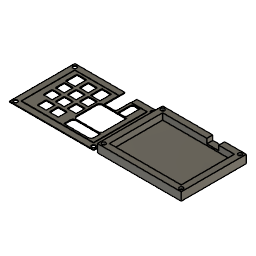
hackpad-case (Autodesk Fusion 360 design; units mm, degrees)
part number: 2026-01-27-21-45-44-218
Autodesk Fusion 360 part; units mm, degrees
sketch "Sketch1" plane through (0, 0, 0) normal (0, 0, 1) x (1, 0, 0)
  line L0 (56.89, -42.155) -> (-56.89, -42.155)
  line L1 (-56.89, -42.155) -> (-56.89, 42.155)
  line L2 (-56.89, 42.155) -> (56.89, 42.155)
  line L3 (56.89, 42.155) -> (56.89, -42.155)
  line L4 (56.89, -42.155) -> (-56.89, 42.155) construction
  line L5 (-56.89, -42.155) -> (56.89, 42.155) construction
  line L6 (66.39, 51.655) -> (-66.39, 51.655)
  line L7 (-66.39, 51.655) -> (-66.39, -51.655)
  line L8 (-66.39, -51.655) -> (66.39, -51.655)
  line L9 (66.39, -51.655) -> (66.39, 51.655)
  line L10 (66.39, 51.655) -> (-66.39, -51.655) construction
  line L11 (-66.39, 51.655) -> (66.39, -51.655) construction
  circle A0 centre (61.39, 46.655) radius 1.7
  circle A1 centre (61.39, -46.655) radius 1.7
  circle A2 centre (-61.39, -46.655) radius 1.7
  circle A3 centre (-61.39, 46.655) radius 1.7
  circle A4 centre (61.39, 46.655) radius 3
  circle A5 centre (61.39, -46.655) radius 3
  circle A6 centre (-61.39, -46.655) radius 3
  circle A7 centre (-61.39, 46.655) radius 3
  dimension "d1" = 113.78
  dimension "d2" = 84.31
  dimension "d7" = 3.4
  dimension "d8" = 5
  dimension "d9" = 5
  dimension "d10" = 9.5
  dimension "d11" = 9.5
  dimension "d12" = 9.5
  dimension "d13" = 3.4
  dimension "d14" = 5
  dimension "d15" = 5
  dimension "d16" = 3.4
  dimension "d17" = 5
  dimension "d18" = 5
  dimension "d19" = 3.4
  dimension "d20" = 5
  dimension "d21" = 5
  dimension "d22" = 6
  dimension "d23" = 6
  dimension "d24" = 6
  dimension "d25" = 6
  constraint horizontal L0
  constraint perpendicular L0 L1
  constraint parallel L0 L2
  constraint parallel L1 L3
  constraint coincident L4 origin
  constraint coincident L5 origin
  constraint horizontal L6
  constraint perpendicular L6 L7
  constraint parallel L6 L8
  constraint parallel L7 L9
  constraint coincident L10 origin
  constraint coincident L11 origin
  constraint concentric A0 A4
  constraint concentric A1 A5
  constraint concentric A2 A6
  constraint concentric A3 A7
  measures "d1" distance of L1.end L2.end
  measures "d2" distance of L0.end L1.end
  measures "d7" diameter of A0
  measures "d8" distance of L9 A0.centre
  measures "d9" distance of L6 A0.centre
  measures "d10" distance of L2 L6
  measures "d11" distance of L0 L8
  measures "d12" distance of L3 L9
  measures "d13" diameter of A1
  measures "d14" distance of L8 A1.centre
  measures "d15" distance of L9 A1.centre
  measures "d16" diameter of A2
  measures "d17" distance of L8 A2.centre
  measures "d18" distance of L7 A2.centre
  measures "d19" diameter of A3
  measures "d20" distance of L6 A3.centre
  measures "d21" distance of L7 A3.centre
  measures "d22" diameter of A4
  measures "d23" diameter of A5
  measures "d24" diameter of A6
  measures "d25" diameter of A7
extrude "Extrude1" add sketch "Sketch1" along normal blind 9.9 from surface at 3.1 contours A4 | A5 | A6 | A7 makes body 1 at (-58.3937, -46.8045, 9.7) makes body 2 at (63.9499, -48.2193, 9.7) makes body 3 at (-63.9499, 48.2193, 9.7) makes body 4 at (58.3937, 46.5055, 9.7)
extrude "Extrude2" add sketch "Sketch1" along normal blind 13 contours L6 L7 L8 L9 bodies 1 2 3 4
extrude "Extrude3" add sketch "Sketch1" along normal blind 3 contours L0 L1 L2 L3 bodies 1
sketch "Sketch2" plane through (0, 0, 13) normal (0, 0, 1) x (-1, 0, 0)
  circle A0 centre (61.39, 46.655) radius 1.7
  circle A1 centre (-61.39, -46.655) radius 1.7
  line L0 (56.89, -42.155) -> (-56.89, -42.155)
  line L1 (-56.89, -42.155) -> (-56.89, 42.155)
  line L2 (-56.89, 42.155) -> (56.89, 42.155)
  line L3 (56.89, 42.155) -> (56.89, -42.155)
  line L4 (-66.39, 51.655) -> (-66.39, -51.655)
  line L5 (-66.39, -51.655) -> (66.39, -51.655)
  line L6 (66.39, -51.655) -> (66.39, 51.655)
  line L7 (66.39, 51.655) -> (-66.39, 51.655)
  circle A2 centre (-61.39, 46.655) radius 1.7
  circle A3 centre (61.39, -46.655) radius 1.7
  line L8 (-12.076, -51.655) -> (-12.076, -42.155)
  line L9 (-30.576, -51.655) -> (-30.576, -42.155)
  line L10 (-66.39, 51.655) -> (-66.39, -51.655)
  line L11 (-56.89, -42.155) -> (-56.89, 42.155)
  dimension "d33" = 18.5
  dimension "d35" = 26.314
  constraint coincident L5 L8.start
  constraint coincident L0 L8.end
  constraint perpendicular L0 L8
  constraint coincident L5 L9.start
  constraint coincident L0 L9.end
  constraint perpendicular L5 L9
  measures "d33" distance of L8 L9
  measures "d35" distance of L9 L11
extrude "Extrude4" cut sketch "Sketch2" against normal blind 7.5 contours L0 L5 L8 L9 bodies 1
sketch "plate-2026-01-28T03_03_28.937Z" plane through (0, 0, 0) normal (0, 0, 1) x (1, 0, 0)
  line L0 (-162.925, -2.525) -> (-149.925, -2.525)
  line L1 (-162.925, -16.525) -> (-149.925, -16.525)
  line L2 (-163.425, -3.025) -> (-163.425, -16.025)
  line L3 (-149.425, -3.025) -> (-149.425, -16.025)
  arc A0 (-162.925, -2.525) -> (-163.425, -3.025) centre (-162.925, -3.025) ccw
  arc A1 (-149.425, -3.025) -> (-149.925, -2.525) centre (-149.925, -3.025) ccw
  arc A2 (-163.425, -16.025) -> (-162.925, -16.525) centre (-162.925, -16.025) ccw
  arc A3 (-149.925, -16.525) -> (-149.425, -16.025) centre (-149.925, -16.025) ccw
  line L4 (-181.975, -21.575) -> (-168.975, -21.575)
  line L5 (-181.975, -35.575) -> (-168.975, -35.575)
  line L6 (-182.475, -22.075) -> (-182.475, -35.075)
  line L7 (-168.475, -22.075) -> (-168.475, -35.075)
  arc A4 (-181.975, -21.575) -> (-182.475, -22.075) centre (-181.975, -22.075) ccw
  arc A5 (-168.475, -22.075) -> (-168.975, -21.575) centre (-168.975, -22.075) ccw
  arc A6 (-182.475, -35.075) -> (-181.975, -35.575) centre (-181.975, -35.075) ccw
  arc A7 (-168.975, -35.575) -> (-168.475, -35.075) centre (-168.975, -35.075) ccw
  line L8 (-162.925, -21.575) -> (-149.925, -21.575)
  line L9 (-162.925, -35.575) -> (-149.925, -35.575)
  line L10 (-163.425, -22.075) -> (-163.425, -35.075)
  line L11 (-149.425, -22.075) -> (-149.425, -35.075)
  arc A8 (-162.925, -21.575) -> (-163.425, -22.075) centre (-162.925, -22.075) ccw
  arc A9 (-149.425, -22.075) -> (-149.925, -21.575) centre (-149.925, -22.075) ccw
  arc A10 (-163.425, -35.075) -> (-162.925, -35.575) centre (-162.925, -35.075) ccw
  arc A11 (-149.925, -35.575) -> (-149.425, -35.075) centre (-149.925, -35.075) ccw
  line L12 (-143.875, -21.575) -> (-130.875, -21.575)
  line L13 (-143.875, -35.575) -> (-130.875, -35.575)
  line L14 (-144.375, -22.075) -> (-144.375, -35.075)
  line L15 (-130.375, -22.075) -> (-130.375, -35.075)
  arc A12 (-143.875, -21.575) -> (-144.375, -22.075) centre (-143.875, -22.075) ccw
  arc A13 (-130.375, -22.075) -> (-130.875, -21.575) centre (-130.875, -22.075) ccw
  arc A14 (-144.375, -35.075) -> (-143.875, -35.575) centre (-143.875, -35.075) ccw
  arc A15 (-130.875, -35.575) -> (-130.375, -35.075) centre (-130.875, -35.075) ccw
  line L16 (-181.975, -40.625) -> (-168.975, -40.625)
  line L17 (-181.975, -54.625) -> (-168.975, -54.625)
  line L18 (-182.475, -41.125) -> (-182.475, -54.125)
  line L19 (-168.475, -41.125) -> (-168.475, -54.125)
  arc A16 (-181.975, -40.625) -> (-182.475, -41.125) centre (-181.975, -41.125) ccw
  arc A17 (-168.475, -41.125) -> (-168.975, -40.625) centre (-168.975, -41.125) ccw
  arc A18 (-182.475, -54.125) -> (-181.975, -54.625) centre (-181.975, -54.125) ccw
  arc A19 (-168.975, -54.625) -> (-168.475, -54.125) centre (-168.975, -54.125) ccw
  line L20 (-162.925, -40.625) -> (-149.925, -40.625)
  line L21 (-162.925, -54.625) -> (-149.925, -54.625)
  line L22 (-163.425, -41.125) -> (-163.425, -54.125)
  line L23 (-149.425, -41.125) -> (-149.425, -54.125)
  arc A20 (-162.925, -40.625) -> (-163.425, -41.125) centre (-162.925, -41.125) ccw
  arc A21 (-149.425, -41.125) -> (-149.925, -40.625) centre (-149.925, -41.125) ccw
  arc A22 (-163.425, -54.125) -> (-162.925, -54.625) centre (-162.925, -54.125) ccw
  arc A23 (-149.925, -54.625) -> (-149.425, -54.125) centre (-149.925, -54.125) ccw
  line L24 (-143.875, -40.625) -> (-130.875, -40.625)
  line L25 (-143.875, -54.625) -> (-130.875, -54.625)
  line L26 (-144.375, -41.125) -> (-144.375, -54.125)
  line L27 (-130.375, -41.125) -> (-130.375, -54.125)
  arc A24 (-143.875, -40.625) -> (-144.375, -41.125) centre (-143.875, -41.125) ccw
  arc A25 (-130.375, -41.125) -> (-130.875, -40.625) centre (-130.875, -41.125) ccw
  arc A26 (-144.375, -54.125) -> (-143.875, -54.625) centre (-143.875, -54.125) ccw
  arc A27 (-130.875, -54.625) -> (-130.375, -54.125) centre (-130.875, -54.125) ccw
  circle A28 centre (-191.875, 4.4557) radius 1.7
  circle A29 centre (-79.875, -81.8599) radius 1.7
  line L28 (-196.875, 10.1401) -> (-196.875, -86.8599)
  line L29 (-196.875, -86.8599) -> (-74.875, -86.8599)
  line L30 (-74.875, -86.8599) -> (-74.875, 9.4557)
  line L31 (-74.875, 9.4557) -> (-109.2354, 9.4557)
  line L32 (-109.2354, -0.0443) -> (-84.2214, -0.0179)
  line L33 (-84.2214, -0.0179) -> (-84.2214, -78.5291)
  line L34 (-84.2214, -78.5291) -> (-187.375, -78.5291)
  line L35 (-187.375, -78.5291) -> (-187.375, -0.0443)
  line L36 (-187.375, -0.0443) -> (-107.2527, -0.0443)
  circle A30 centre (-79.875, 4.4557) radius 1.7
  circle A31 centre (-191.875, -81.8599) radius 1.7
  line L37 (-187.375, -0.0443) -> (-187.375, -78.5291)
  line L38 (-187.375, -78.5291) -> (-84.2214, -78.5291)
  line L39 (-84.2214, -78.5291) -> (-84.2214, -0.0179)
  line L40 (-196.875, 9.4557) -> (-109.2354, 9.4557)
  line L41 (-109.2354, -0.0443) -> (-107.2527, -0.0443)
  circle A32 centre (-191.875, 4.4557) radius 3
  circle A33 centre (-191.875, -81.8599) radius 3
  circle A34 centre (-79.875, -81.8599) radius 3
  circle A35 centre (-79.875, 4.4557) radius 3
  line L42 (-123.3934, -26.7131) -> (-85.9914, -26.7131)
  line L43 (-85.9914, -26.7131) -> (-85.9914, -53.0661)
  line L44 (-89.9914, -57.0661) -> (-122.3934, -57.0661)
  line L45 (-127.3934, -52.0661) -> (-127.3934, -30.7131)
  line L46 (-124.3934, -61.2571) -> (-85.9914, -61.2571)
  line L47 (-85.9914, -61.2571) -> (-85.9914, -70.3221)
  line L48 (-88.9914, -73.3221) -> (-127.3934, -73.3221)
  line L49 (-127.3934, -73.3221) -> (-127.3934, -64.2571)
  line L50 (-196.875, 10.1401) -> (-196.875, 9.4557)
  arc A36 (-127.3934, -52.0661) -> (-122.3934, -57.0661) centre (-122.3934, -52.0661) ccw
  line L51 (-123.3934, -26.7131) -> (-127.3934, -30.7131)
  line L52 (-85.9914, -53.0661) -> (-89.9914, -57.0661)
  line L53 (-127.3934, -64.2571) -> (-124.3934, -61.2571)
  line L54 (-85.9914, -70.3221) -> (-88.9914, -73.3221)
  line L55 (-98.0014, -2.3043) -> (-92.2714, -2.3043)
  line L56 (-90.2714, -4.3043) -> (-90.2714, -23.1243)
  line L57 (-90.2714, -23.1243) -> (-98.0014, -23.1243)
  line L58 (-100.0014, -21.1243) -> (-100.0014, -4.3043)
  line L59 (-121.1354, -0.3901) -> (-105.3354, -0.3901)
  line L60 (-105.3354, -0.3901) -> (-105.3354, -19.6081)
  line L61 (-107.3354, -21.6081) -> (-120.1354, -21.6081)
  line L62 (-123.1354, -18.6081) -> (-123.1354, -2.3901)
  line L63 (-119.2354, -0.0268) -> (-119.2354, 9.4557)
  line L64 (-109.2354, -0.0443) -> (-109.2354, 9.4557)
  arc A37 (-121.1354, -0.3901) -> (-123.1354, -2.3901) centre (-121.1354, -2.3901) ccw
  arc A38 (-107.3354, -21.6081) -> (-105.3354, -19.6081) centre (-107.3354, -19.6081) ccw
  arc A39 (-90.2714, -4.3043) -> (-92.2714, -2.3043) centre (-92.2714, -4.3043) ccw
  arc A40 (-100.0014, -21.1243) -> (-98.0014, -23.1243) centre (-98.0014, -21.1243) ccw
  line L65 (-123.1354, -18.6081) -> (-123.1354, -21.6081)
  line L66 (-123.1354, -21.6081) -> (-120.1354, -21.6081)
  line L67 (-98.0014, -2.3043) -> (-100.0014, -2.3043)
  line L68 (-100.0014, -2.3043) -> (-100.0014, -4.3043)
  line L69 (-119.2354, -0.0268) -> (-119.2354, -0.3901)
  line L70 (-109.2354, -0.0443) -> (-109.2354, -0.3901)
  point P0 (-79.875, -81.8599)
  point P1 (-190.0693, -81.8599)
  point P2 (-190.0693, 5.1401)
  point P3 (-78.0693, 5.1401)
  point P4 (-127.3934, -26.7131)
  point P5 (-85.9914, -57.0661)
  point P6 (-127.3934, -57.0661)
  point P7 (-127.3934, -61.2571)
  point P8 (-85.9914, -73.3221)
  point P9 (-100.0014, -2.3043)
  point P10 (-90.2714, -2.3043)
  point P11 (-100.0014, -23.1243)
  point P12 (-123.1354, -0.3901)
  point P13 (-123.1354, -21.6081)
  dimension "d44" = 5.05
  dimension "d53" = 6
  dimension "d54" = 6
  dimension "d55" = 6
  dimension "d56" = 6
  dimension "d57" = 9.5
  dimension "d63" = 97
  dimension "d64" = 9.5
  dimension "d65" = 9.5
  dimension "d66" = 4.9
  dimension "d71" = 30.353
  dimension "d72" = 12.065
  dimension "d73" = 1.77
  dimension "d74" = 1.77
  dimension "d75" = 41.402
  dimension "d76" = 41.402
  dimension "d77" = 4.191
  dimension "d78" = 5.207
  dimension "d79" = 3.4
  dimension "d80" = 5
  dimension "d81" = 5
  dimension "d83" = 122
  dimension "d84" = 5
  dimension "d85" = 5
  dimension "d86" = 5
  dimension "d87" = 5
  dimension "d88" = 5
  dimension "d89" = 3.4
  dimension "d90" = 5
  dimension "d91" = 5
  dimension "d93" = 4
  dimension "d94" = 4
  dimension "d95" = 4
  dimension "d96" = 3
  dimension "d97" = 3
  dimension "d98" = 3
  dimension "d99" = 3
  dimension "d100" = 9.73
  dimension "d101" = 20.82
  dimension "d102" = 6.05
  dimension "d103" = 2.28
  dimension "d104" = 17.8
  dimension "d105" = 21.218
  dimension "d106" = 5.334
  dimension "d107" = 0.35
  dimension "d109" = 10
  dimension "d110" = 3.9
  dimension "d111" = 3.9
  dimension "d112" = 2
  dimension "d113" = 2
  dimension "d114" = 2
  dimension "d115" = 3
  dimension "d116" = 3
  dimension "d117" = 2
  dimension "d118" = 2
  constraint parallel L31 L40
  constraint parallel L36 L41
  constraint concentric A28 A32
  constraint concentric A31 A33
  constraint coincident P0 A29.centre
  constraint concentric A30 A35
  constraint vertical L39
  constraint horizontal L42
  constraint vertical L43
  constraint horizontal L44
  constraint vertical L45
  constraint horizontal L46
  constraint vertical L47
  constraint horizontal L48
  constraint vertical L49
  constraint perpendicular L40 L50
  constraint horizontal L29
  constraint vertical L30
  constraint horizontal L31
  constraint horizontal L34
  constraint concentric A29 A34
  constraint coincident P6 L45
  constraint coincident P6 L44
  constraint tangent L45 A36
  constraint tangent L44 A36
  constraint coincident P4 L42
  constraint coincident P4 L45
  constraint coincident P5 L43
  constraint coincident P5 L44
  constraint coincident P7 L49
  constraint coincident P7 L46
  constraint coincident P8 L47
  constraint coincident P8 L48
  constraint horizontal L55
  constraint vertical L56
  constraint horizontal L57
  constraint vertical L58
  constraint horizontal L59
  constraint vertical L60
  constraint horizontal L61
  constraint vertical L62
  constraint coincident L40 L63.end
  constraint perpendicular L40 L63
  constraint coincident P12 L59
  constraint coincident P12 L62
  constraint tangent L59 A37
  constraint tangent L62 A37
  constraint tangent L60 A38
  constraint tangent L61 A38
  constraint coincident P10 L55
  constraint coincident P10 L56
  constraint tangent L55 A39
  constraint tangent L56 A39
  constraint coincident P11 L57
  constraint coincident P11 L58
  constraint tangent L57 A40
  constraint tangent L58 A40
  constraint equal A39 A40
  constraint coincident P13 L62
  constraint coincident P13 L61
  constraint coincident P9 L55
  constraint coincident P9 L58
  constraint coincident P13 L65.end
  constraint coincident P9 L67.end
  constraint coincident L59 L69.end
  constraint perpendicular L59 L69
  constraint coincident L59 L70.end
  constraint perpendicular L59 L70
  measures "d44" distance of L9 L20
  measures "d53" diameter of A32
  measures "d54" diameter of A33
  measures "d55" diameter of A34
  measures "d56" diameter of A35
  measures "d57" distance of L31.end L32.start
  measures "d63" distance of L28.start L28.end
  measures "d64" distance of L28 L37
  measures "d65" distance of L40 L41
  measures "d66" distance of L6 L37
  measures "d71" distance of P4 P6
  measures "d72" distance of P7 L48.end
  measures "d73" distance of L39 L43
  measures "d74" distance of L33 L47
  measures "d75" distance of P8 L48.end
  measures "d76" distance of P5 P6
  measures "d77" distance of L44 L46
  measures "d78" vertical distance of L33.end P8
  measures "d79" diameter of A31
  measures "d80" distance of L28 A31.centre
  measures "d81" distance of L29 A31.centre
  measures "d83" distance of L28.end L29.end
  measures "d84" distance of A28.centre L40
  measures "d85" distance of A28.centre L28
  measures "d86" distance of L31 A30.centre
  measures "d87" distance of L30 A30.centre
  measures "d88" distance of P0 L30
  measures "d89" diameter of A29
  measures "d90" distance of P0 L29
  measures "d91" radius of A36
  measures "d93" distance of P4 L45.end
  measures "d94" distance of P5 L43.end
  measures "d95" distance of P5 L44.start
  measures "d96" distance of P7 L49.end
  measures "d97" distance of P7 L46.start
  measures "d98" distance of P8 L47.end
  measures "d99" distance of P8 L48.start
  measures "d100" distance of P9 P10
  measures "d101" distance of P9 P11
  measures "d102" distance of L33 L56
  measures "d103" distance of L32 P10
  measures "d104" distance of P12 L59.end
  measures "d105" distance of P12 P13
  measures "d106" distance of L58 L60
  measures "d107" distance of L32 L59.end
  measures "d109" horizontal distance of L32.start L63.start
  measures "d110" horizontal distance of L32.start L59.end
  measures "d111" horizontal distance of P12 L63.start
  measures "d112" radius of A37
  measures "d113" radius of A38
  measures "d114" radius of A39
  measures "d115" distance of P13 L62.start
  measures "d116" distance of P13 L61.end
  measures "d117" distance of P9 L55.start
  measures "d118" distance of P9 L58.end
extrude "Extrude7" add 1 faces at (24.4093, 45.3217, 5.5) along direction (0, 0, 1) blind 7.5 on bodies 1 bodies 1
other "Base Mesh Feature1"
sketch "Sketch4" plane through (0, 0, 13) normal (0, 0, 1) x (-1, 0, 0)
  line L0 (56.89, -42.155) -> (-56.89, -42.155)
  line L1 (-56.89, -42.155) -> (-56.89, 42.155)
  line L2 (-56.89, 42.155) -> (56.89, 42.155)
  line L3 (56.89, 42.155) -> (56.89, -42.155)
  circle A0 centre (61.39, -46.655) radius 1.7
  circle A1 centre (-61.39, 46.655) radius 1.7
  line L4 (-66.39, -51.655) -> (66.39, -51.655)
  line L5 (66.39, -51.655) -> (66.39, 51.655)
  line L6 (66.39, 51.655) -> (-66.39, 51.655)
  line L7 (-66.39, 51.655) -> (-66.39, -51.655)
  circle A2 centre (-61.39, -46.655) radius 1.7
  circle A3 centre (61.39, 46.655) radius 1.7
  line L8 (56.89, -42.155) -> (-56.89, -42.155)
  line L9 (-56.89, -42.155) -> (-56.89, 42.155)
  line L10 (-56.89, 42.155) -> (56.89, 42.155)
  line L11 (56.89, 42.155) -> (56.89, -42.155)
  circle A4 centre (61.39, -46.655) radius 1.7
  circle A5 centre (61.39, -46.655) radius 3
  circle A6 centre (61.39, 46.655) radius 1.7
  circle A7 centre (61.39, 46.655) radius 3
  circle A8 centre (-61.39, 46.655) radius 1.7
  circle A9 centre (-61.39, 46.655) radius 3
  circle A10 centre (-61.39, -46.655) radius 1.7
  circle A11 centre (-61.39, -46.655) radius 3
  dimension "d125" = 6
  dimension "d126" = 6
  dimension "d127" = 6
  dimension "d128" = 6
  constraint horizontal L8
  constraint vertical L9
  constraint horizontal L10
  constraint vertical L11
  constraint coincident L1.end L2.start
  constraint coincident L0.start L3.end
  constraint concentric A0 A4
  constraint concentric A4 A5
  constraint concentric A3 A6
  constraint concentric A6 A7
  constraint concentric A1 A8
  constraint concentric A8 A9
  constraint concentric A2 A10
  constraint concentric A10 A11
  measures "d125" diameter of A5
  measures "d126" diameter of A7
  measures "d127" diameter of A9
  measures "d128" diameter of A11
sketch "plate-2026-01-28T03_03_28.937Z (1)" plane through (0, 0, 13) normal (0, 0, 1) x (1, 0, 0)
  line L0 (111.5924, 36.2585) -> (124.5924, 36.2585)
  line L1 (111.5924, 22.2585) -> (124.5924, 22.2585)
  line L2 (111.0924, 35.7585) -> (111.0924, 22.7585)
  line L3 (125.0924, 35.7585) -> (125.0924, 22.7585)
  arc A0 (111.5924, 36.2585) -> (111.0924, 35.7585) centre (111.5924, 35.7585) ccw
  arc A1 (125.0924, 35.7585) -> (124.5924, 36.2585) centre (124.5924, 35.7585) ccw
  arc A2 (111.0924, 22.7585) -> (111.5924, 22.2585) centre (111.5924, 22.7585) ccw
  arc A3 (124.5924, 22.2585) -> (125.0924, 22.7585) centre (124.5924, 22.7585) ccw
  line L4 (92.5424, 17.2085) -> (105.5424, 17.2085)
  line L5 (92.5424, 3.2085) -> (105.5424, 3.2085)
  line L6 (92.0424, 16.7085) -> (92.0424, 3.7085)
  line L7 (106.0424, 16.7085) -> (106.0424, 3.7085)
  arc A4 (92.5424, 17.2085) -> (92.0424, 16.7085) centre (92.5424, 16.7085) ccw
  arc A5 (106.0424, 16.7085) -> (105.5424, 17.2085) centre (105.5424, 16.7085) ccw
  arc A6 (92.0424, 3.7085) -> (92.5424, 3.2085) centre (92.5424, 3.7085) ccw
  arc A7 (105.5424, 3.2085) -> (106.0424, 3.7085) centre (105.5424, 3.7085) ccw
  line L8 (111.5924, 17.2085) -> (124.5924, 17.2085)
  line L9 (111.5924, 3.2085) -> (124.5924, 3.2085)
  line L10 (111.0924, 16.7085) -> (111.0924, 3.7085)
  line L11 (125.0924, 16.7085) -> (125.0924, 3.7085)
  arc A8 (111.5924, 17.2085) -> (111.0924, 16.7085) centre (111.5924, 16.7085) ccw
  arc A9 (125.0924, 16.7085) -> (124.5924, 17.2085) centre (124.5924, 16.7085) ccw
  arc A10 (111.0924, 3.7085) -> (111.5924, 3.2085) centre (111.5924, 3.7085) ccw
  arc A11 (124.5924, 3.2085) -> (125.0924, 3.7085) centre (124.5924, 3.7085) ccw
  line L12 (130.6424, 17.2085) -> (143.6424, 17.2085)
  line L13 (130.6424, 3.2085) -> (143.6424, 3.2085)
  line L14 (130.1424, 16.7085) -> (130.1424, 3.7085)
  line L15 (144.1424, 16.7085) -> (144.1424, 3.7085)
  arc A12 (130.6424, 17.2085) -> (130.1424, 16.7085) centre (130.6424, 16.7085) ccw
  arc A13 (144.1424, 16.7085) -> (143.6424, 17.2085) centre (143.6424, 16.7085) ccw
  arc A14 (130.1424, 3.7085) -> (130.6424, 3.2085) centre (130.6424, 3.7085) ccw
  arc A15 (143.6424, 3.2085) -> (144.1424, 3.7085) centre (143.6424, 3.7085) ccw
  line L16 (92.5424, -1.8415) -> (105.5424, -1.8415)
  line L17 (92.5424, -15.8415) -> (105.5424, -15.8415)
  line L18 (92.0424, -2.3415) -> (92.0424, -15.3415)
  line L19 (106.0424, -2.3415) -> (106.0424, -15.3415)
  arc A16 (92.5424, -1.8415) -> (92.0424, -2.3415) centre (92.5424, -2.3415) ccw
  arc A17 (106.0424, -2.3415) -> (105.5424, -1.8415) centre (105.5424, -2.3415) ccw
  arc A18 (92.0424, -15.3415) -> (92.5424, -15.8415) centre (92.5424, -15.3415) ccw
  arc A19 (105.5424, -15.8415) -> (106.0424, -15.3415) centre (105.5424, -15.3415) ccw
  line L20 (111.5924, -1.8415) -> (124.5924, -1.8415)
  line L21 (111.5924, -15.8415) -> (124.5924, -15.8415)
  line L22 (111.0924, -2.3415) -> (111.0924, -15.3415)
  line L23 (125.0924, -2.3415) -> (125.0924, -15.3415)
  arc A20 (111.5924, -1.8415) -> (111.0924, -2.3415) centre (111.5924, -2.3415) ccw
  arc A21 (125.0924, -2.3415) -> (124.5924, -1.8415) centre (124.5924, -2.3415) ccw
  arc A22 (111.0924, -15.3415) -> (111.5924, -15.8415) centre (111.5924, -15.3415) ccw
  arc A23 (124.5924, -15.8415) -> (125.0924, -15.3415) centre (124.5924, -15.3415) ccw
  line L24 (130.6424, -1.8415) -> (143.6424, -1.8415)
  line L25 (130.6424, -15.8415) -> (143.6424, -15.8415)
  line L26 (130.1424, -2.3415) -> (130.1424, -15.3415)
  line L27 (144.1424, -2.3415) -> (144.1424, -15.3415)
  arc A24 (130.6424, -1.8415) -> (130.1424, -2.3415) centre (130.6424, -2.3415) ccw
  arc A25 (144.1424, -2.3415) -> (143.6424, -1.8415) centre (143.6424, -2.3415) ccw
  arc A26 (130.1424, -15.3415) -> (130.6424, -15.8415) centre (130.6424, -15.3415) ccw
  arc A27 (143.6424, -15.8415) -> (144.1424, -15.3415) centre (143.6424, -15.3415) ccw
  line L28 (121.2182, -34.8915) -> (134.2185, -34.8915)
  arc A28 (134.2185, -34.8915) -> (134.7185, -34.3915) centre (134.2185, -34.3915) ccw
  arc A29 (134.7185, -21.3915) -> (134.2185, -20.8915) centre (134.2185, -21.3915) ccw
  arc A30 (120.6174, -34.3915) -> (121.2182, -34.8915) centre (121.1587, -34.352) ccw
  arc A31 (121.2182, -20.8915) -> (120.6174, -21.3914) centre (121.1587, -21.4309) ccw
  line L29 (120.6174, -21.3914) -> (120.6174, -34.3915)
  line L30 (134.7185, -21.3915) -> (134.7185, -34.3915)
  line L31 (121.2182, -20.8915) -> (134.2185, -20.8915)
  line L32 (114.9665, -34.8915) -> (101.9662, -34.8915)
  arc A32 (115.5674, -21.3914) -> (114.9665, -20.8915) centre (115.026, -21.4309) ccw
  line L33 (101.4662, -21.3915) -> (101.4662, -34.3915)
  line L34 (114.9665, -20.8915) -> (101.9662, -20.8915)
  arc A33 (101.9662, -20.8915) -> (101.4662, -21.3915) centre (101.9662, -21.3915) ccw
  arc A34 (114.9665, -34.8915) -> (115.5674, -34.3915) centre (115.026, -34.352) ccw
  line L35 (115.5674, -21.3914) -> (115.5674, -34.3915)
  arc A35 (101.4662, -34.3915) -> (101.9662, -34.8915) centre (101.9662, -34.3915) ccw
  circle A36 centre (61.39, 46.655) radius 1.7
  circle A37 centre (61.39, -46.655) radius 1.7
  line L36 (-56.89, 42.155) -> (56.89, 42.155)
  dimension "d130" = 5.05
  dimension "d134" = 5.05
  dimension "d135" = 5.8965
  measures "d130" distance of L21 L31
  measures "d134" distance of L29 L35
  measures "d135" distance of L0 L36
sketch "Sketch6" plane through (0, 0, 13) normal (0, 0, 1) x (1, 0, 0)
  line L0 (197.7016, -41.9833) -> (83.1186, -41.9833)
  line L1 (83.1186, -41.9833) -> (83.1186, 42.8484)
  line L2 (83.1186, 42.8484) -> (197.7016, 42.8484)
  line L3 (197.7016, 42.8484) -> (197.7016, -41.9833)
  line L4 (153.1976, -24.3309) -> (191.1976, -24.3309)
  line L5 (191.1976, -24.3309) -> (191.1976, -34.3309)
  line L6 (186.1976, -39.3309) -> (148.1976, -39.3309)
  line L7 (148.1976, -39.3309) -> (148.1976, -29.3309)
  line L8 (150.6321, 17.4739) -> (190.6321, 17.4739)
  line L9 (190.6321, 17.4739) -> (190.6321, -20.5261)
  line L10 (187.6321, -23.5261) -> (152.6321, -23.5261)
  line L11 (147.6321, -18.5261) -> (147.6321, 14.4739)
  line L12 (179, 41) -> (188, 41)
  line L13 (188, 41) -> (188, 21.5)
  line L14 (185, 18.5) -> (176, 18.5)
  line L15 (176, 18.5) -> (176, 38)
  line L16 (153.3081, 42.8484) -> (172, 42.8484)
  line L17 (172, 42.8484) -> (172, 22)
  line L18 (169, 19) -> (153.3081, 19)
  line L19 (153.3081, 19) -> (153.3081, 42.8484)
  arc A0 (147.6321, -18.5261) -> (152.6321, -23.5261) centre (152.6321, -18.5261) ccw
  line L20 (150.6321, 17.4739) -> (147.6321, 14.4739)
  line L21 (190.6321, -20.5261) -> (187.6321, -23.5261)
  arc A1 (186.1976, -39.3309) -> (191.1976, -34.3309) centre (186.1976, -34.3309) ccw
  arc A2 (153.1976, -24.3309) -> (148.1976, -29.3309) centre (153.1976, -29.3309) ccw
  arc A3 (169, 19) -> (172, 22) centre (169, 22) ccw
  arc A4 (179, 41) -> (176, 38) centre (179, 38) ccw
  arc A5 (185, 18.5) -> (188, 21.5) centre (185, 21.5) ccw
  line L22 (130.3424, 38.6085) -> (145.3424, 38.6085)
  line L23 (145.3424, 38.6085) -> (145.3424, 20.6085)
  line L24 (145.3424, 20.6085) -> (130.3424, 20.6085)
  line L25 (130.3424, 20.6085) -> (130.3424, 38.6085)
  line L26 (125.0924, 35.7585) -> (125.0924, 22.7585)
  line L27 (130.6424, 17.2085) -> (143.6424, 17.2085)
  line L28 (105.8424, 20.6085) -> (90.8424, 20.6085)
  line L29 (90.8424, 38.6085) -> (105.8424, 38.6085)
  line L30 (105.8424, 38.6085) -> (105.8424, 20.6085)
  line L31 (90.8424, 20.6085) -> (90.8424, 38.6085)
  line L32 (111.0924, 35.7585) -> (111.0924, 22.7585)
  line L33 (92.5424, 17.2085) -> (105.5424, 17.2085)
  line L34 (73.6186, 52.3484) -> (207.2016, 52.3484)
  line L35 (207.2016, 52.3484) -> (207.2016, -51.4833)
  line L36 (207.2016, -51.4833) -> (73.6186, -51.4833)
  line L37 (73.6186, -51.4833) -> (73.6186, 52.3484)
  circle A6 centre (78.6186, 47.3484) radius 1.7
  circle A7 centre (78.6186, 47.3484) radius 3
  circle A8 centre (78.6186, -46.4833) radius 1.7
  circle A9 centre (78.6186, -46.4833) radius 3
  circle A10 centre (202.2016, -46.4833) radius 1.7
  circle A11 centre (202.2016, -46.4833) radius 3
  circle A12 centre (202.2016, 47.3484) radius 1.7
  circle A13 centre (202.2016, 47.3484) radius 3
  line L38 (155.0325, 42.8484) -> (155.0325, 52.3484)
  line L39 (170.0325, 52.3484) -> (170.0325, 42.8484)
  point P0 (147.6321, 17.4739)
  point P1 (190.6321, -23.5261)
  dimension "d136" = 5
  dimension "d137" = 3
  dimension "d138" = 3
  dimension "d139" = 3
  dimension "d140" = 3
  dimension "d141" = 5
  dimension "d142" = 3
  dimension "d143" = 3
  dimension "d144" = 41
  dimension "d145" = 43
  dimension "d146" = 43
  dimension "d147" = 15
  dimension "d148" = 15
  dimension "d149" = 18
  dimension "d150" = 5.25
  dimension "d151" = 3.4
  dimension "d152" = 15
  dimension "d153" = 18
  dimension "d154" = 5.25
  dimension "d155" = 3.4
  dimension "d156" = 9.5
  dimension "d157" = 9.5
  dimension "d158" = 9.5
  dimension "d159" = 9.5
  dimension "d160" = 3.4
  dimension "d161" = 6
  dimension "d162" = 5
  dimension "d163" = 5
  dimension "d164" = 3.4
  dimension "d165" = 6
  dimension "d166" = 5
  dimension "d167" = 5
  dimension "d168" = 3.4
  dimension "d169" = 6
  dimension "d170" = 5
  dimension "d171" = 5
  dimension "d172" = 3.4
  dimension "d173" = 6
  dimension "d174" = 5
  dimension "d175" = 5
  dimension "d177" = 15
  constraint horizontal L0
  constraint vertical L1
  constraint horizontal L2
  constraint vertical L3
  constraint horizontal L4
  constraint vertical L5
  constraint horizontal L6
  constraint vertical L7
  constraint horizontal L8
  constraint vertical L9
  constraint horizontal L10
  constraint vertical L11
  constraint horizontal L12
  constraint vertical L13
  constraint horizontal L14
  constraint vertical L15
  constraint horizontal L16
  constraint vertical L17
  constraint horizontal L18
  constraint vertical L19
  constraint coincident L2 L16.start
  constraint tangent L10 A0
  constraint tangent L11 A0
  constraint coincident P0 L8
  constraint coincident P0 L11
  constraint coincident P1 L9
  constraint coincident P1 L10
  constraint tangent L5 A1
  constraint tangent L6 A1
  constraint tangent L4 A2
  constraint tangent L7 A2
  constraint equal A1 A2
  constraint tangent L17 A3
  constraint tangent L18 A3
  constraint tangent L12 A4
  constraint tangent L15 A4
  constraint tangent L13 A5
  constraint tangent L14 A5
  constraint equal A4 A5
  constraint horizontal L22
  constraint vertical L23
  constraint horizontal L24
  constraint vertical L25
  constraint horizontal L29
  constraint vertical L30
  constraint horizontal L28
  constraint vertical L31
  constraint horizontal L34
  constraint vertical L35
  constraint horizontal L36
  constraint vertical L37
  constraint concentric A6 A7
  constraint concentric A8 A9
  constraint concentric A10 A11
  constraint concentric A12 A13
  constraint coincident L2 L38.start
  constraint coincident L34 L38.end
  constraint perpendicular L34 L38
  constraint coincident L34 L39.start
  constraint coincident L2 L39.end
  constraint perpendicular L2 L39
  measures "d136" radius of A0
  measures "d137" distance of P0 L8.start
  measures "d138" distance of P0 L11.end
  measures "d139" distance of P1 L9.end
  measures "d140" distance of P1 L10.start
  measures "d141" radius of A1
  measures "d142" radius of A3
  measures "d143" radius of A4
  measures "d144" distance of L8.end P1
  measures "d145" distance of L9 L11
  measures "d146" distance of L5 L7
  measures "d147" distance of L4 L6
  measures "d148" distance of L22.start L22.end
  measures "d149" distance of L22.start L24.end
  measures "d150" distance of L25 L26
  measures "d151" distance of L24 L27
  measures "d152" distance of L29.start L29.end
  measures "d153" distance of L28.end L29.start
  measures "d154" distance of L30 L32
  measures "d155" distance of L28 L33
  measures "d156" distance of L2 L34
  measures "d157" distance of L0 L36
  measures "d158" distance of L1 L37
  measures "d159" distance of L3 L35
  measures "d160" diameter of A6
  measures "d161" diameter of A7
  measures "d162" distance of L34 A6.centre
  measures "d163" distance of L37 A6.centre
  measures "d164" diameter of A8
  measures "d165" diameter of A9
  measures "d166" distance of L36 A8.centre
  measures "d167" distance of L37 A8.centre
  measures "d168" diameter of A10
  measures "d169" diameter of A11
  measures "d170" distance of L35 A10.centre
  measures "d171" distance of L36 A10.centre
  measures "d172" diameter of A12
  measures "d173" diameter of A13
  measures "d174" distance of L34 A12.centre
  measures "d175" distance of L35 A12.centre
  measures "d177" distance of L38 L39
extrude "Extrude8" add sketch "Sketch6" along normal blind 1 separate body contours L0 L1 L2 L3 L16 L34 L35 L36 L37 L38 L39 makes body 5
extrude "Extrude9" add sketch "Sketch6" along normal blind 1.5 contours L0 L1 L2 L3 L17 L18 L19 A3 bodies 5
extrude "Extrude10" cut sketch "plate-2026-01-28T03_03_28.937Z (1)" along normal blind 15 contours L0 L1 L2 L3 A0 A1 A2 A3 | L4 L5 L6 L7 A4 A5 A6 A7 | L8 L9 L10 L11 A8 A9 A10 A11 | L12 L13 L14 L15 A12 A13 A14 A15 | L16 L17 L18 L19 A16 A17 A18 A19 | L20 L21 L22 L23 A20 A21 A22 A23 | L24 L25 L26 L27 A24 A25 A26 A27 | L28 A28 A29 A30 A31 L29 L30 L31 | L32 A32 L33 L34 A33 A34 L35 A35 bodies 5
extrude "Extrude11" add sketch "Sketch4" against normal blind 9.9 from surface at -3.1 separate body contours A5 | A7 | A9 | A11 makes body 6 at (63.9499, -45.0907, 3.3) makes body 7 at (63.9499, 48.2193, 3.3) makes body 8 at (-64.3863, -46.5055, 3.3) makes body 9 at (-63.9499, 45.0907, 3.3)
extrude "Extrude12" add sketch "Sketch1" along normal blind 13 separate body contours L6 L7 L8 L9 makes body 10
extrude "Extrude14" add sketch "Sketch1" along normal blind 3 contours L0 L1 L2 L3 bodies 10
move_body "Move1" bodies 5 to x (1, 0, 0) y (0, 1, 0) z (0, 0, 1) at (-140, 0, 0)
sketch "Sketch7" plane through (0, 51.655, 0) normal (0, 1, 0) x (-1, 0, 0)
  line L0 (66.39, 13) -> (-66.39, 13)
  line L1 (-66.39, 13) -> (-66.39, 0)
  line L2 (-66.39, 0) -> (66.39, 0)
  line L3 (66.39, 0) -> (66.39, 13)
  line L4 (-32, 13) -> (-32, 5.5)
  line L5 (-13.2947, 14.4148) -> (-13.2947, 5.5)
  line L6 (-13.2947, 5.5) -> (-32, 5.5)
  line L7 (-32, 14.5) -> (-32, 13)
  line L8 (-32, 14.5) -> (-13.2947, 14.4148)
  constraint coincident L0 L4.start
  constraint perpendicular L0 L4
  constraint perpendicular L4 L6
  constraint perpendicular L0 L7
extrude "Extrude15" cut sketch "Sketch7" along normal blind -23 and the other way blind -3 contours L0 L5 L7 L8 | L0 L4 L5 L6 bodies 5 10
move_body "Move2" bodies 5 to x (1, 0, 0) y (0, 1, 0) z (0, 0, 1) at (-140, 0, -13)
hidden bodies 1
equation "d35 = 20.564 mm + 5.75 mm"
equation "d92 = 4.00 mm"
equation "d93 = d92"
equation "d95 = d94"
equation "d97 = d96"
equation "d99 = d98"
equation "d116 = d115"
equation "d118 = d117"
equation "d138 = d137"
equation "d140 = d139"
